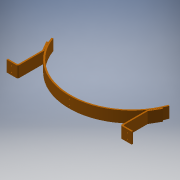
# Autodesk Inventor part: Half moon catch
Saved by Autodesk Inventor 2017 (Build 210142000, 142)
## iProperties
Created: 2017-01-15
Part Number: Half moon catch
Material: Generic
Document SubType Name: Modeling
Designer: Ben
Density: 1 g/cm^3
Appearance: Orange
Author: Ben
Autodesk Inventor part; units mm, degrees
ref_plane "YZ Plane" through (0, 0, 0) normal (1, 0, 0) x (0, 1, 0)
ref_plane "XZ Plane" through (0, 0, 0) normal (0, 1, 0) x (-1, 0, 0)
ref_plane "XY Plane" through (0, 0, 0) normal (0, 0, 1) x (1, 0, 0)
sketch "Sketch1" plane through (0, 0, 0) normal (0, 1, 0) x (-1, 0, 0)
  arc A0 (131.275059, 47.780214) -> (-131.275059, 47.780214) centre (0, 0) ccw
  arc A1 (134.258583, 48.866128) -> (-134.258583, 48.866128) centre (0, 0) ccw
  line L0 (150.393801, 142.875) -> (-175.785181, 142.875) construction
  line L1 (0, 0) -> (131.275059, 47.780214) construction
  line L2 (0, 0) -> (-131.275059, 47.780214) construction
  line L3 (0, 0) -> (0, 139.7) construction
  line L4 (-131.275059, 47.780214) -> (-134.258583, 48.866128)
  line L5 (131.275059, 47.780214) -> (134.258583, 48.866128)
  line L6 (130.08338, 60.438977) -> (116.95801, 83.172784)
  line L7 (116.95801, 83.172784) -> (116.95801, 142.875)
  line L8 (116.95801, 142.875) -> (142.35801, 142.875)
  line L9 (142.35801, 139.7) -> (142.35801, 142.875)
  line L10 (142.35801, 139.7) -> (120.13301, 139.7)
  line L11 (120.13301, 139.7) -> (120.13301, 84.023523)
  line L12 (120.13301, 84.023523) -> (132.83301, 62.026477)
  line L13 (132.83301, 62.026477) -> (130.08338, 60.438977)
  line L14 (120.13301, 139.7) -> (116.95801, 139.7) construction
  line L15 (123.73338, 71.4375) -> (126.48301, 73.025) construction
  line L16 (-130.08338, 60.438977) -> (-116.95801, 83.172784)
  line L17 (-116.95801, 83.172784) -> (-116.95801, 142.875)
  line L18 (-116.95801, 142.875) -> (-142.35801, 142.875)
  line L19 (-142.35801, 139.7) -> (-142.35801, 142.875)
  line L20 (-142.35801, 139.7) -> (-120.13301, 139.7)
  line L21 (-120.13301, 139.7) -> (-120.13301, 84.023523)
  line L22 (-120.13301, 84.023523) -> (-132.83301, 62.026477)
  line L23 (-132.83301, 62.026477) -> (-130.08338, 60.438977)
  dimension "d1" = 3.175
  dimension "d4" = 279.4
  dimension "d6" = 140
  dimension "d7" = 3.175
  dimension "d8" = 25.4
  dimension "d9" = 30
  dimension "d10" = 25.4
  constraints: 48 end point, 8 symmetric about line, 6 perpendicular, 6 point on circle, 4 coincident, 4 point on line, 2 centre point, 2 collinear, 2 equal length, 2 horizontal, 2 tangent, 1 midpoint, 1 parallel, 1 vertical
  measures "d1" distance of L5.end L1.end
  measures "d4" diameter of A0
  measures "d6" angle of L1 L2
  measures "d7" distance of L9.start L8.end
  measures "d8" distance of L7.end L8.end
  measures "d9" angle of L7 L6
  measures "d10" distance of L11.end L12.end
extrude "Extrusion1" add sketch "Sketch1" along normal blind 25.4
fillet "Fillet1" radius 3.175 4 edges at (-120.133, 12.7, 139.7) (-116.958, 12.7, 142.875) (116.958, 12.7, 142.875) (120.133, 12.7, 139.7)
sketch "Sketch2" plane through (-142.35801, 0, 142.875) normal (0, 0, 1) x (1, 0, 0)
  line L0 (142.35801, 0) -> (142.35801, 0) construction
  circle A0 centre (9.00801, 19.05) radius 1.5875
  circle A1 centre (142.35801, 19.05) radius 1.5875
  circle A2 centre (275.70801, 19.05) radius 1.5875
  line L1 (11.082951, 0) -> (11.082951, 0) construction
  line L2 (142.35801, 0) -> (142.35801, 25.4) construction
  line L3 (266.09139, 25.4) -> (18.624631, 25.4) construction
  line L4 (275.70801, 19.05) -> (9.00801, 19.05) construction
  line L5 (275.70801, 12.7) -> (9.00801, 12.7) construction
  circle A3 centre (9.00801, 6.35) radius 1.5875
  circle A4 centre (142.35801, 6.35) radius 1.5875
  circle A5 centre (275.70801, 6.35) radius 1.5875
  line L6 (9.00801, 19.05) -> (9.00801, 6.35) construction
  line L7 (275.70801, 19.05) -> (275.70801, 6.35) construction
  line L8 (0, 0) -> (0, 25.4) construction
  line L9 (9.00801, 12.7) -> (0, 12.7) construction
  point P0 (11.082951, 25.4)
  dimension "d13" = 3.175
  dimension "d22" = 12.7
  dimension "d23" = 266.7
  constraints: 16 end point, 6 centre point, 5 midpoint, 4 vertical, 3 symmetric about line, 2 coincident, 2 equal radius, 2 horizontal, 2 point on line, 4 other
  measures "d13" diameter of A2
  measures "d22" distance from line of A4.centre L4
  measures "d23" distance between parallel lines of L7 L6
extrude "Extrusion2" cut sketch "Sketch2" against normal blind 25.4
body "Solid1"
